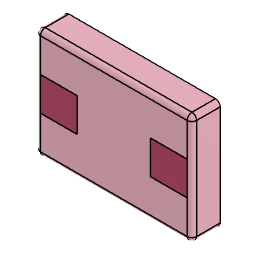
nose_plate (Autodesk Fusion 360 design; units mm, degrees)
part number: 2025-10-11-08-44-41-819
Autodesk Fusion 360 part; units mm, degrees
note: some values were not read from the file. Set by a fixed rule: which sketch regions a step uses.
sketch "Nose Plate" plane through (0, 0, 0) normal (0, 1, 0) x (1, 0, 0)
  line L0 (0, 0) -> (66, 0)
  line L1 (66, 0) -> (66, -46.5)
  line L2 (66, -46.5) -> (0, -46.5)
  line L3 (0, -46.5) -> (0, 0)
  dimension "d5" = 66
  dimension "d6" = 46.5
  constraint horizontal L0
  constraint vertical L1
  constraint horizontal L2
  constraint vertical L3
  constraint coincident L0.start L3.end
  measures "d5" distance of L0.start L0.end
  measures "d6" distance of L0.start L2.end
extrude "Extrude1" add sketch "Nose Plate" along normal blind 12 makes body 1
sketch "Nostrils" plane through (0, 0, 0) normal (0, -1, 0) x (1, 0, 0)
  line L0 (66, 46.5) -> (0, 46.5)
  line L1 (0, 46.5) -> (0, 0)
  line L2 (0, 0) -> (66, 0)
  line L3 (66, 0) -> (66, 46.5)
  line L4 (2, 30.3333) -> (17.5, 30.3333)
  line L5 (17.5, 30.3333) -> (17.5, 16.1667)
  line L6 (17.5, 16.1667) -> (2, 16.1667)
  line L7 (2, 16.1667) -> (2, 30.3333)
  line L8 (48.5, 30.3333) -> (64, 30.3333)
  line L9 (64, 30.3333) -> (64, 16.1667)
  line L10 (64, 16.1667) -> (48.5, 16.1667)
  line L11 (48.5, 16.1667) -> (48.5, 30.3333)
  dimension "d22" = 15.5
  dimension "d23" = 15.5
  dimension "d24" = 31
  dimension "d25" = 14.1667
  dimension "d26" = 14.1667
  dimension "d27" = 16.1667
  dimension "d28" = 16.1667
  dimension "d39" = 2
  dimension "d40" = 2
  constraint horizontal L4
  constraint vertical L5
  constraint horizontal L6
  constraint vertical L7
  constraint horizontal L8
  constraint vertical L9
  constraint horizontal L10
  constraint vertical L11
  measures "d22" distance of L4.start L4.end
  measures "d23" distance of L8.start L8.end
  measures "d24" distance of L5 L11
  measures "d25" distance of L4 L6
  measures "d26" distance of L8 L10
  measures "d27" distance of L0 L4
  measures "d28" distance of L0 L8
  measures "d39" distance of L1 L7
  measures "d40" distance of L3 L9
extrude "Extrude4" add sketch "Nostrils" along normal blind 0.01 separate body contours L4 L5 L6 L7 | L8 L9 L10 L11 makes body 2 at (7.1667, 0, 25.6111) makes body 3 at (53.6667, 0, 20.8889)
fillet "Fillet1" radius 2 8 edges at (0, 6, 46.5) (0, 0, 23.25) (33, 0, 46.5) (66, 6, 46.5) (66, 0, 23.25) (66, 6, 0) (33, 0, 0) (0, 6, 0) on bodies 1
equation "block_size = 16 mm" comment "The size of the blocks used for the dimensions of the Minecraft Pig."
equation "pine_thickness = 12 mm" comment "The thickness of the pine boards used for the Minecraft Pig's body."
equation "nose_plate_height = 3 * face_block_height" comment "The height of the Nose Plate that makes up the Minecraft Pig's face."
equation "nose_plate_width = 4 * face_block_width" comment "The width of the Nose Plate that makes up the Minecraft Pig's face."
equation "d5 = nose_plate_width"
equation "d6 = nose_plate_height"
equation "d7 = pine_thickness"
equation "nostril_block_width = ( nose_plate_width - 2 * fillet_radius ) / 4" comment "The width of the blocks used for the Minecraft Pig's nostrils."
equation "d22 = nostril_block_width"
equation "d23 = nostril_block_width"
equation "d25 = nostril_block_height"
equation "d26 = nostril_block_height"
equation "d27 = nostril_block_height + fillet_radius"
equation "d28 = nostril_block_height + fillet_radius"
equation "front_face_plate_height = 8 * block_size" comment "The height of the Front Face Plate that makes up the Minecraft Pig's face."
equation "front_face_plate_width = 10 * block_size - 2 * pine_thickness" comment "The width of the Front Face Plate that makes up the Minecraft Pig's face."
equation "face_block_width = ( front_face_plate_width - 2 * fillet_radius ) / 8" comment "The width of the blocks used for the Minecraft Pig's eyes."
equation "fillet_radius = 2 mm" comment "The radius of the fillets applied to the Front Face Plate."
equation "face_block_height = ( front_face_plate_height - 2 * fillet_radius ) / 8" comment "The height of the blocks used for the Minecraft Pig's eyes."
equation "nostril_block_height = ( nose_plate_height - 2 * fillet_radius ) / 3" comment "The height of the blocks used for the Minecraft Pig's nostrils."
equation "d39 = fillet_radius"
equation "d40 = fillet_radius"
equation "d44 = fillet_radius"
named bodies: "Nose Plate", "Right Nostril", "Left Nostril"
